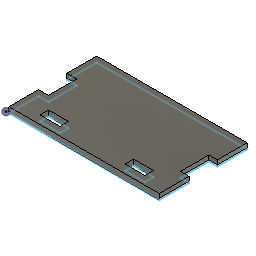
holder (Autodesk Fusion 360 design; units mm, degrees)
Autodesk Fusion 360 part; units mm, degrees
sketch "Sketch1" plane through (0, 0, 0) normal (0, 0, 1) x (1, 0, 0) in component "Component"
  line L0 (1, 10.4524) -> (4.5037, 10.4512)
  line L1 (4.5037, 10.4512) -> (4.5073, 20.4512)
  line L2 (4.5073, 20.4512) -> (1.0073, 20.4524)
  line L3 (1.0073, 20.4524) -> (1.011, 30.9524)
  line L4 (54, 31) -> (54, 20.5)
  line L5 (54, 20.5) -> (51, 20.5)
  line L6 (51, 20.5) -> (51, 10.5)
  line L7 (51, 10.5) -> (54, 10.5)
  line L8 (54, 10.5) -> (54, 0)
  line L9 (46, 3) -> (46, 6)
  line L10 (9, 6) -> (9, 3)
  line L11 (39, 6) -> (39, 3)
  line L12 (16, 6) -> (16, 3)
  line L13 (1, 10.4524) -> (0.9963, 0.0409)
  line L14 (1.011, 30.9524) -> (54, 31)
  line L15 (0.9963, 0.0409) -> (54, 0)
  line L16 (39, 6) -> (46, 6)
  line L17 (46, 3) -> (39, 3)
  line L18 (16, 3) -> (9, 3)
  line L19 (9, 6) -> (16, 6)
  dimension "d2" = 10
  dimension "d3" = 10.5
  dimension "d5" = 10.5
  dimension "d6" = 10
  dimension "d7" = 10.5
  constraint perpendicular L0 L1
  constraint perpendicular L1 L2
  constraint perpendicular L2 L3
  constraint perpendicular L4 L5
  constraint perpendicular L5 L6
  constraint perpendicular L6 L7
  constraint perpendicular L7 L8
  constraint perpendicular L0 L13
  constraint vertical L12
  constraint vertical L10
  constraint vertical L11
  constraint vertical L9
  constraint perpendicular L9 L16
  constraint perpendicular L11 L17
  constraint perpendicular L10 L18
  constraint perpendicular L12 L19
  measures "d2" distance of L0.end L1.end
  measures "d3" distance of L2.end L3.end
  measures "d5" distance of L4.start L4.end
  measures "d6" distance of L5.end L6.end
  measures "d7" distance of L7.end L8.end
sketch "Sketch1 (2)" plane through (0, 0, 0) normal (0, 0, 1) x (1, 0, 0) in component "Component'"
  arc A0 (0, 0) -> (0, 80) centre (-30, 40) ccw
  arc A1 (55, 80) -> (55, 0) centre (85, 40) ccw
  line L0 (0, 80) -> (0, 87.6963)
  line L1 (55, 80) -> (55, 87.6963)
  line L2 (0, 80) -> (-2, 80)
  line L3 (0, 87.6963) -> (-2, 87.6963)
  line L4 (-2, 87.6963) -> (-2, 80)
  line L5 (-2, 80) -> (-2, 87.6963)
  arc A2 (-2, 80) -> (-2, 87.6963) centre (-0.9371, 83.8481) ccw
  arc A3 (-2, 80) -> (-2, 87.6963) centre (-0.9371, 83.8481) ccw
  arc A4 (55.1257, 87.6963) -> (55.1257, 80) centre (54.0629, 83.8481) ccw
  arc A5 (-2, 87.6963) -> (55, 87.6963) centre (26.5, 119.7443) ccw
  line L6 (0, 0) -> (15, 0)
  line L7 (15, 0) -> (15, -2)
  line L8 (15, -2) -> (0, -2)
  line L9 (0, -2) -> (0, 0)
  line L10 (55, 0) -> (41, 0)
  line L11 (41, 0) -> (41, -2)
  line L12 (41, -2) -> (55, -2)
  line L13 (55, -2) -> (55, 0)
  arc A6 (15, 0) -> (0, 5) centre (3.5, -9.5) ccw
  line L14 (0, 5) -> (0, 0)
  line L15 (55, 0) -> (55, 5)
  arc A7 (55, 5) -> (41, 0) centre (51, -5.9) ccw
  spline S0 degree 2 poles (15, 0) (27, 33) (41, 0) knots 0 0 0 5.592865 5.592865 5.592865 weights 1 3 1
  constraint coincident A0.start L6.start
  constraint vertical L0
  constraint perpendicular L0 L2
  constraint perpendicular L0 L3
  constraint perpendicular L2 L4
  constraint horizontal L6
  constraint vertical L7
  constraint horizontal L8
  constraint vertical L9
  constraint horizontal L10
  constraint vertical L11
  constraint horizontal L12
  constraint vertical L13
  constraint perpendicular L6 L14
  constraint perpendicular L10 L15
extrude "Extrude1" add sketch "Sketch1 (2)" along normal blind 2 makes body 1 in component "Component'"
extrude "Extrude2" add sketch "Sketch1 (2)" along normal blind 16 separate body contours A0 A6 L14 | A0 L6 A6 | L6 L7 L8 L9 makes body 2 in component "Component'"
extrude "Extrude3" cut sketch "Sketch1 (2)" along normal blind 14 contours A0 A6 L14 | A0 L6 A6 | L6 L7 L8 L9 bodies 1 2 in component "Component'"
extrude "Extrude4" add sketch "Sketch1 (2)" along normal blind 2 contours A0 A6 L14 | A0 L6 A6 | L6 L7 L8 L9 bodies 1 in component "Component'"
extrude "Extrude5" cut sketch "Sketch1 (2)" along normal blind 16 contours L6 L7 L8 L9 bodies 1 2 in component "Component'"
extrude "Extrude6" add sketch "Sketch1 (2)" along normal blind 16 contours L6 L7 L8 L9 bodies 1 2 in component "Component'"
extrude "Extrude7" cut sketch "Sketch1 (2)" along normal blind 16 contours A0 L0 A2 A3 A5 | L0 L2 L4 L5 A5 | L0 L3 A2 A3 A5 | L0 L3 A5 bodies 1 in component "Component'"
extrude "Extrude8" add sketch "Sketch1 (2)" along normal blind 16 contours A0 L0 A2 A3 A5 | L0 L2 L4 L5 A5 | L0 L3 A2 A3 A5 | L0 L3 A5 bodies 1 in component "Component'"
extrude "Extrude9" cut sketch "Sketch1 (2)" along normal blind 14 contours A0 L0 A2 A3 A5 | L0 L2 L4 L5 A5 | L0 L3 A2 A3 A5 | L0 L3 A5 bodies 1 makes body 3 at (-1.3333, 82.5654, 16) in component "Component'"
extrude "Extrude10" add sketch "Sketch1 (2)" along normal blind 2 contours A0 L0 A2 A3 A5 | L0 L2 L4 L5 A5 | L0 L3 A2 A3 A5 | L0 L3 A5 bodies 1 in component "Component'"
extrude "Extrude11" cut sketch "Sketch1 (2)" along normal blind 16 contours L0 L2 L4 L5 A5 | L0 L3 A5 bodies 1 3 in component "Component'"
extrude "Extrude12" add sketch "Sketch1 (2)" along normal blind 16 contours L0 L2 L4 L5 A5 | L0 L3 A5 bodies 1 3 in component "Component'"
fillet "Fillet1" radius 0.5 tangency weight 1.51342 1 edges at (-2, 83.8481, 16) on bodies 1 in component "Component'"
fillet "Fillet2" radius 0.5 1 edges at (7.5, -2, 16) on bodies 1 in component "Component'"
fillet "Fillet3" radius 0.5 1 edges at (7.5, -2, 0) on bodies 1 in component "Component'"
fillet "Fillet4" radius 0.5 1 edges at (-2, 83.8481, 0) on bodies 1 in component "Component'"
fillet "Fillet5" radius 0.5 1 edges at (19.8457, 43.9257, 2) on bodies 1 in component "Component'"
extrude "Extrude2'" add sketch "Sketch1" along normal blind 2 separate body makes body 4 in component "Component"
fillet "Fillet1'" radius 0.5 11 edges at (54, 5.25, 0) (52.5, 10.5, 0) (51, 15.5, 0) (52.5, 20.5, 0) (54, 25.75, 0) (27.5055, 30.9762, 0) (1.0091, 25.7024, 0) (4.5055, 15.4512, 0) (2.7573, 20.4518, 0) (2.7519, 10.4518, 0) (0.9982, 5.2467, 0) on bodies 4 in component "Component"
component "Component" placed x (1, 0, 0) y (0, 1, 0) z (0, 0, 1) at (0, 0, 0)
component "Component'" placed x (1, 0, 0) y (0, 1, 0) z (0, 0, 1) at (0, 0, 0)
